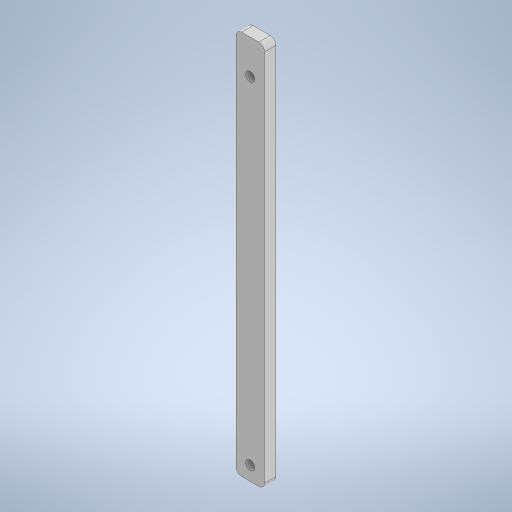
# Autodesk Inventor part: BP_BOX-Bar-add
Saved by Autodesk Inventor 2024.3 (Build 283343000, 343)
## iProperties
Created: 2025-10-31
Part Number: BP_BOX-Bar-add
Material: 一般
Document SubType Name: Modeling
Designer: 佐藤智貴
Density: 1 g/cm^3
Appearance: 既定
Author: 佐藤智貴
Autodesk Inventor part; units mm, degrees
ref_plane "YZ Plane" through (0, 0, 0) normal (1, 0, 0) x (0, 1, 0)
ref_plane "XZ Plane" through (0, 0, 0) normal (0, 1, 0) x (-1, 0, 0)
ref_plane "XY Plane" through (0, 0, 0) normal (0, 0, 1) x (1, 0, 0)
sketch "スケッチ1" plane through (0, 0, 0) normal (0, 0, 1) x (1, 0, 0)
  line L0 (0, 0) -> (10, 0)
  line L1 (10, 0) -> (10, 135)
  line L2 (10, 135) -> (0, 135)
  line L3 (0, 135) -> (0, 0)
  dimension "d0" = 10
  dimension "d1" = 135
  constraints: 8 end point, 2 parallel, 1 horizontal, 1 perpendicular
  measures "d0" distance of L1.end L2.end
  measures "d1" distance of L0.end L1.end
extrude "押し出し1" add sketch "スケッチ1" along normal blind 4
sketch "スケッチ2" plane through (0, 0, 4) normal (0, 0, 1) x (1, 0, 0)
  line L0 (10, 135) -> (0, 135) projected
  line L1 (10, 0) -> (10, 135) projected
  point P0 (0, 0)
  point P1 (5, 123)
  point P2 (5, 5)
  dimension "d4" = 12
  dimension "d5" = 5
  dimension "d14" = 118
  measures "d4" distance from line of L0 point (5, 123)
  measures "d5" distance from line of L1 point (5, 123)
  measures "d14" distance of point (5, 123) point (5, 5)
hole "穴1" at (5, 123, 4) at (5, 5, 4) direction (0, 0, -1) diameter 3.2 end through all
fillet "フィレット1" radius 2 4 edges at (0, 135, 2) (0, 0, 2) (10, 135, 2) (10, 0, 2)
